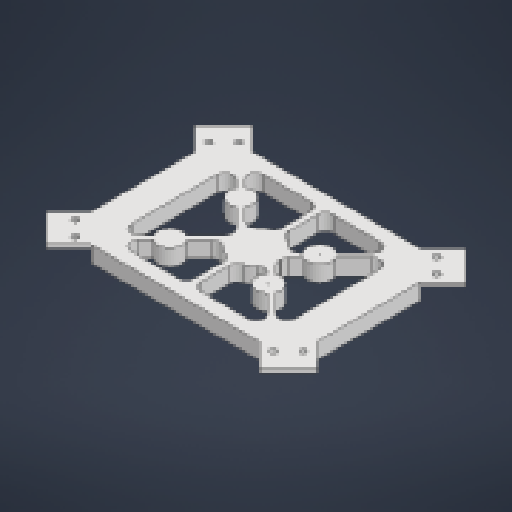
# Autodesk Inventor part: Base
Saved by Autodesk Inventor 2023 (Build 270158000, 158)
## iProperties
Created: 2023-01-21
Part Number: Base
Material: Generic
Document SubType Name: Modeling
Designer: Michael
Density: 1 g/cm^3
Appearance: Default
Author: Michael
Autodesk Inventor part; units mm, degrees
ref_plane "YZ Plane" through (0, 0, 0) normal (1, 0, 0) x (0, 1, 0)
ref_plane "XZ Plane" through (0, 0, 0) normal (0, 1, 0) x (-1, 0, 0)
ref_plane "XY Plane" through (0, 0, 0) normal (0, 0, 1) x (1, 0, 0)
sketch "Sketch1" plane through (0, 0, 0) normal (0, 1, 0) x (-1, 0, 0)
  line L0 (0, 0) -> (177.8, 0)
  line L1 (177.8, 0) -> (177.8, -127)
  line L2 (177.8, -127) -> (0, -127)
  line L3 (0, -127) -> (0, 0)
  line L4 (155.3506, 0) -> (177.8, -22.4519) projected
  line L5 (173.3121, 17.9595) -> (155.3506, 0) projected
  line L6 (195.7615, -4.4923) -> (173.3121, 17.9595) projected
  line L7 (177.8, -22.4519) -> (195.7615, -4.4923) projected
  line L8 (195.7615, -122.5077) -> (177.8, -104.5481) projected
  line L9 (173.3121, -144.9595) -> (195.7615, -122.5077) projected
  line L10 (155.3506, -127) -> (173.3121, -144.9595) projected
  line L11 (177.8, -104.5481) -> (155.3506, -127) projected
  line L12 (22.4494, 0) -> (4.4879, 17.9595) projected
  line L13 (0, -22.4519) -> (22.4494, 0) projected
  line L14 (4.4879, 17.9595) -> (-17.9615, -4.4923) projected
  line L15 (-17.9615, -4.4923) -> (0, -22.4519) projected
  line L16 (22.4494, -127) -> (0, -104.5481) projected
  line L17 (4.4879, -144.9595) -> (22.4494, -127) projected
  line L18 (0, -104.5481) -> (-17.9615, -122.5077) projected
  line L19 (-17.9615, -122.5077) -> (4.4879, -144.9595) projected
  circle A0 centre (178.6987, -10.7776) radius 2.4765
  circle A1 centre (167.025, 0.8974) radius 2.4765
  circle A2 centre (178.6987, -116.2224) radius 2.4765
  circle A3 centre (167.025, -127.8974) radius 2.4765
  circle A4 centre (10.775, -127.8974) radius 2.4765
  circle A5 centre (-0.8987, -116.2224) radius 2.4765
  circle A6 centre (-0.8987, -10.7776) radius 2.4765
  circle A7 centre (10.775, 0.8974) radius 2.4765
  dimension "d0" = 177.8
  dimension "d1" = 127
  constraints: 8 centre point, 8 end point, 2 parallel, 1 horizontal, 1 perpendicular, 16 other
  measures "d0" distance of L1.end L2.end
  measures "d1" distance of L0.end L1.end
extrude "Extrusion1" add sketch "Sketch1" along normal blind 12.7 contours L13 L3 A6 L0 A7 | L0 A7 L3 A6 L15 L14 L12 | L0 L4 L1 L11 L2 L16 L3 L13 | L5 L6 L7 L1 A0 L0 A1 | L0 A1 L1 A0 L4 | L16 L2 A4 L3 A5 | L3 A5 L2 A4 L17 L19 L18 | L8 L9 L10 L2 A3 L1 A2 | L1 A2 L2 A3 L11
sketch "Sketch6" plane through (0, 12.7, 0) normal (0, 1, 0) x (1, 0, 0)
  line L0 (-165.1, 5.1549) -> (-12.7, 5.1549)
  line L1 (-12.7, 5.1549) -> (-12.7, 121.9349)
  line L2 (-12.7, 121.9349) -> (-165.1, 121.9349)
  line L3 (-165.1, 121.9349) -> (-165.1, 5.1549)
  line L4 (-177.8, 104.5481) -> (-177.8, 22.4519) projected
  line L5 (0, 22.4519) -> (0, 104.5481) projected
  line L6 (0, 63.5) -> (-177.8, 63.5)
  line L7 (-22.4494, 127) -> (-155.3506, 127) projected
  line L8 (-88.9, 127) -> (-88.9, 0)
  point P0 (-203.2, 129.9481)
  point P1 (-203.2, 22.4519)
  point P2 (-180.7506, 0)
  point P3 (-22.4494, 0)
  point P4 (-177.8, 127)
  point P5 (-177.8, 0)
  point P6 (-127, 91.5035)
  point P7 (-127, 35.5035)
  point P8 (-57, 43.5035)
  point P9 (-57, 83.5035)
  dimension "d38" = 152.4
  dimension "d39" = 116.7799
  dimension "d78" = 12.7
  dimension "d80" = 56
  dimension "d81" = 28.0035
  dimension "d82" = 70
  dimension "d83" = 70
  dimension "d84" = 40
  dimension "d85" = 38.1
  constraints: 12 end point, 3 midpoint, 2 parallel, 1 horizontal, 1 perpendicular, 1 vertical
  measures "d38" distance of L2.end L1.end
  measures "d39" distance of L1.end L0.end
  measures "d78" distance between parallel lines of L3 L4
  measures "d80" distance of point (-127, 91.503) point (-127, 35.504)
  measures "d81" distance from line of point (-127, 91.503) L6
  measures "d82" horizontal distance of point (-57, 83.504) point (-127, 91.503)
  measures "d83" horizontal distance of point (-57, 43.504) point (-127, 35.504)
  measures "d84" distance of point (-57, 83.504) point (-57, 43.504)
  measures "d85" distance from line of point (-127, 91.503) L8
hole "Hole1" at (-127, 12.7, -91.5035) at (-127, 12.7, -35.5035) at (-57, 12.7, -43.5035) at (-57, 12.7, -83.5035) direction (0, -1, 0) diameter 2.4 end through all
sketch "Sketch11" plane through (0, 12.7, 0) normal (0, 1, 0) x (1, 0, 0)
  circle A0 centre (-57, 43.5035) radius 1.2 projected
  circle A1 centre (-127, 91.5035) radius 1.2 projected
  circle A2 centre (-127, 35.5035) radius 1.2 projected
  circle A3 centre (-57, 83.5035) radius 1.2 projected
  line L0 (-195.7615, 4.4923) -> (-173.3121, -17.9595) projected
  line L1 (-173.3121, -17.9595) -> (-155.3506, 0) projected
  line L2 (-155.3506, 0) -> (-22.4494, 0) projected
  line L3 (-22.4494, 0) -> (-4.4879, -17.9595) projected
  line L4 (-4.4879, -17.9595) -> (17.9615, 4.4923) projected
  line L5 (17.9615, 4.4923) -> (0, 22.4519) projected
  line L6 (0, 22.4519) -> (0, 104.5481) projected
  line L7 (0, 104.5481) -> (17.9615, 122.5077) projected
  line L8 (17.9615, 122.5077) -> (-4.4879, 144.9595) projected
  line L9 (-4.4879, 144.9595) -> (-22.4494, 127) projected
  line L10 (-22.4494, 127) -> (-155.3506, 127) projected
  line L11 (-155.3506, 127) -> (-173.3121, 144.9595) projected
  line L12 (-173.3121, 144.9595) -> (-195.7615, 122.5077) projected
  line L13 (-195.7615, 122.5077) -> (-177.8, 104.5481) projected
  line L14 (-177.8, 104.5481) -> (-177.8, 22.4519) projected
  line L15 (-177.8, 22.4519) -> (-195.7615, 4.4923) projected
  circle A4 centre (-167.025, -0.8974) radius 2.4765 projected
  circle A5 centre (-178.6987, 10.7776) radius 2.4765 projected
  circle A6 centre (-178.6987, 116.2224) radius 2.4765 projected
  circle A7 centre (-167.025, 127.8974) radius 2.4765 projected
  circle A8 centre (-10.775, -0.8974) radius 2.4765 projected
  circle A9 centre (0.8987, 10.7776) radius 2.4765 projected
  circle A10 centre (0.8987, 116.2224) radius 2.4765 projected
  circle A11 centre (-10.775, 127.8974) radius 2.4765 projected
  line L16 (-177.8, 63.5) -> (-169.5015, 63.5)
  circle A12 centre (-127, 91.5035) radius 1.2 projected
  circle A13 centre (-127, 91.5035) radius 6.35
  circle A14 centre (-57, 43.5035) radius 1.2 projected
  circle A15 centre (-57, 43.5035) radius 6.35
  circle A16 centre (-57, 83.5035) radius 6.35
  line L17 (-161.925, 15.875) -> (-15.875, 15.875)
  line L18 (-15.875, 111.125) -> (-161.925, 111.125)
  line L19 (-161.925, 111.125) -> (-161.925, 15.875)
  line L20 (-88.9, 0) -> (-88.9, 8.3011)
  line L21 (-15.8748, 83.5035) -> (-31.7498, 83.5035)
  line L22 (-15.8748, 43.4965) -> (-31.7498, 43.4965)
  arc A17 (-31.7498, 83.5035) -> (-31.7498, 43.4965) centre (-0.101, 63.5) ccw
  line L23 (-15.875, 87.3135) -> (-31.75, 87.3135)
  line L24 (-31.75, 91.1235) -> (-15.875, 91.1235)
  arc A18 (-31.75, 91.1235) -> (-31.75, 87.3135) centre (-31.75, 89.2185) ccw
  arc A19 (-15.875, 87.3135) -> (-15.875, 91.1235) centre (-15.875, 89.2185) ccw
  line L25 (-15.8748, 43.4965) -> (-15.8748, 83.5035)
  line L26 (-15.875, 39.6865) -> (-31.75, 39.6865)
  line L27 (-31.75, 35.8765) -> (-15.875, 35.8765)
  arc A20 (-31.75, 39.6865) -> (-31.75, 35.8765) centre (-31.75, 37.7815) ccw
  arc A21 (-15.875, 35.8765) -> (-15.875, 39.6865) centre (-15.875, 37.7815) ccw
  circle A22 centre (-57, 83.5035) radius 1.2 projected
  line L28 (-57, 43.5035) -> (-57, 83.5035)
  line L29 (-22.4494, 127) -> (-155.3506, 127) projected
  line L30 (-127, 35.5035) -> (-118.0302, 44.4732)
  line L31 (-127, 35.5035) -> (-114.3149, 35.5035) construction
  line L32 (-92.075, 60.325) -> (-117.475, 60.325)
  line L33 (-92.075, 60.325) -> (-92.075, 34.925)
  line L34 (-88.9, 8.3011) -> (-88.9, 127)
  line L35 (-169.5015, 63.5) -> (-60.5009, 63.5)
  arc A23 (-92.075, 34.925) -> (-117.475, 60.325) centre (-128.5345, 23.8655) ccw
  line L36 (-92.075, 66.675) -> (-117.475, 66.675)
  line L37 (-92.075, 66.675) -> (-92.075, 92.075)
  arc A24 (-117.475, 66.675) -> (-92.075, 92.075) centre (-128.5345, 103.1345) ccw
  line L38 (-85.725, 60.325) -> (-60.325, 60.325)
  line L39 (-85.725, 60.325) -> (-85.725, 34.925)
  arc A25 (-60.325, 60.325) -> (-85.725, 34.925) centre (-49.2655, 23.8655) ccw
  arc A26 (-85.725, 92.075) -> (-60.325, 66.675) centre (-49.2655, 103.1345) ccw
  line L40 (-85.725, 66.675) -> (-60.325, 66.675)
  line L41 (-85.725, 66.675) -> (-85.725, 92.075)
  line L42 (-127, 60.325) -> (-158.75, 60.325)
  line L43 (-92.075, 30.7686) -> (-92.075, 19.1212)
  line L44 (-143.4535, 19.05) -> (-158.75, 19.05)
  line L45 (-158.75, 19.05) -> (-158.75, 60.325)
  arc A27 (-127, 41.8535) -> (-131.4901, 31.0134) centre (-127, 35.5035) ccw
  arc A28 (-120.65, 35.5035) -> (-123.825, 41.0028) centre (-127, 35.5035) ccw
  line L46 (-131.4901, 31.0134) -> (-143.4535, 19.05)
  line L47 (-127, 41.8535) -> (-127, 60.325)
  line L48 (-92.075, 19.1212) -> (-136.493, 19.1212)
  line L49 (-128.6435, 29.3699) -> (-138.8922, 19.1212)
  line L50 (-128.6435, 29.3699) -> (-114.1497, 29.3699) construction
  line L51 (-138.8922, 19.1212) -> (-136.493, 19.1212)
  arc A29 (-128.6435, 29.3699) -> (-122.5099, 39.9936) centre (-127, 35.5035) ccw
  arc A30 (-127, 41.8535) -> (-131.4901, 31.0134) centre (-127, 35.5035) ccw
  line L52 (-123.825, 60.3251) -> (-123.825, 41.0028)
  arc A31 (-92.075, 24.9449) -> (-123.825, 60.3251) centre (-131.5726, 21.4362) ccw
  point P0 (0, 0)
  point P1 (-88.9, 111.125)
  point P2 (-101.5938, 50.8062)
  point P3 (-101.2536, 47.6312)
  dimension "d104" = 12.7
  dimension "d105" = 12.7
  dimension "d106" = 12.7
  dimension "d107" = 15.875
  dimension "d109" = 15.875
  dimension "d111" = 15.875
  dimension "d112" = 15.875
  dimension "d113" = 15.875
  dimension "d114" = 3.81
  dimension "d115" = 3.81
  dimension "d120" = 45
  dimension "d121" = 25.4
  dimension "d122" = 25.4
  dimension "d123" = 38.1
  dimension "d124" = 3.175
  dimension "d125" = 3.175
  dimension "d127" = 3.175
  dimension "d128" = 3.175
  dimension "d130" = 3.175
  dimension "d131" = 135
  dimension "d133" = 3.175
  dimension "d135" = 0
  dimension "d136" = 0
  dimension "d137" = 3.175
  constraints: 72 end point, 30 point on circle, 18 symmetric about line, 17 centre point, 12 horizontal, 6 vertical, 5 coincident, 5 midpoint, 4 parallel, 4 perpendicular, 4 tangent, 3 point on line, 2 equal length, 7 other
  measures "d104" diameter of A13
  measures "d105" diameter of A15
  measures "d106" diameter of A16
  measures "d107" distance between parallel lines of L19 L14
  measures "d109" distance between parallel lines of L2 L17
  measures "d111" distance of L21.start L21.end
  measures "d112" distance of L22.start L22.end
  measures "d113" distance of L24.end L24.start
  measures "d114" distance of L23.end L24.start
  measures "d115" distance between parallel lines of L23 L21
  measures "d120" angle of L31 L30
  measures "d121" distance of L32.start L32.end
  measures "d122" distance of L32.start L33.end
  measures "d123" radius of A23
  measures "d124" distance between parallel lines of L33 L34
  measures "d125" distance between parallel lines of L35 L32
  measures "d127" distance between parallel lines of L44 L17
  measures "d128" distance between parallel lines of L19 L45
  measures "d130" vertical distance of point (-101.594, 50.806) point (-101.254, 47.631)
  measures "d131" angle of L49 L50
  measures "d133" distance between parallel lines of L46 L49
  measures "d135" distance between parallel lines of L42 L32
  measures "d136" distance from line of A31.start L33
  measures "d137" distance between parallel lines of L52 L47
extrude "Extrusion12" cut sketch "Sketch11" against normal blind 17.4625 contours L33 A23 L32 | L47 A27 L46 L44 L45 L42 | L43 L48 L51 L49 A29 A28 L52 A31
body "Solid1"
